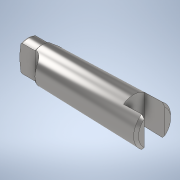
# Autodesk Inventor part: Part005.Morse 5 shaft
Saved by Autodesk Inventor 2022.2 (Build 262287010, 287A)
## iProperties
Created: 2022-11-30
Part Number: Part005.Morse 5 shaft
Material: Steel, Alloy
Document SubType Name: Modeling
Designer: User
Mass: 1240.36 g
Surface Area: 217.832 cm^2
Volume: 160.46 cm^3
Density: 7.73 g/cm^3
Appearance: Semi-Polished
Author: User
Autodesk Inventor part; units mm, degrees
ref_plane "YZ Plane" through (0, 0, 0) normal (1, 0, 0) x (0, 1, 0)
ref_plane "XZ Plane" through (0, 0, 0) normal (0, 1, 0) x (-1, 0, 0)
ref_plane "XY Plane" through (0, 0, 0) normal (0, 0, 1) x (1, 0, 0)
sketch "Sketch1" plane through (0, 0, 0) normal (0, 0, 1) x (1, 0, 0)
  line L0 (0, 0) -> (0, 18.2735) construction
  line L1 (0, 18.2735) -> (20.5646, 18.8146) construction
  line L2 (155.5, 22.3653) -> (155.5, 0)
  line L3 (155.5, 0) -> (0, 0)
  line L4 (149.2, 22.1995) -> (149.2, 0) construction
  line L5 (0, 0) -> (2.3398, 16.0387)
  line L6 (4.3188, 17.75) -> (19.5, 17.75)
  line L7 (19.5, 17.75) -> (20.5646, 18.8146)
  arc A0 (4.3188, 17.75) -> (2.3398, 16.0387) centre (4.3188, 15.75) ccw
  line L8 (20.5646, 18.8146) -> (155.5, 22.3653)
  dimension "d0" = 36.547
  dimension "d1" = 155.5
  dimension "d2" = 44.399
  dimension "d3" = 149.2
  dimension "d4" = 35.5
  dimension "d5" = 45
  dimension "d6" = 19.5
  dimension "d7" = 2
  dimension "d8" = 8.3
  constraints: 18 end point, 3 point on line, 2 parallel, 2 point on circle, 2 tangent, 1 centre point, 1 horizontal, 1 perpendicular, 1 vertical
  measures "d0" diameter of L0.end L3
  measures "d1" distance of L2.end L0.start
  measures "d2" diameter of L4.start L3
  measures "d3" distance between parallel lines of L0 L4
  measures "d4" diameter of L6 L3
  measures "d5" angle of L6 L7
  measures "d6" distance from line of L0 L6.end
  measures "d7" radius of A0
  measures "d8" angle of L5 L0
revolve "Revolution1" add sketch "Sketch1" angle 360 about axis through (155.5, 0, 0) along (-1, 0, 0)
sketch "Sketch2" plane through (0, 0, 0) normal (0, 1, 0) x (-1, 0, 0)
  line L0 (0, 7.95) -> (-19.5007, 7.95)
  arc A0 (-24.5298, 28.7331) -> (-19.5007, 7.95) centre (-19.5007, 18.95) ccw
  line L1 (-24.5298, 28.7331) -> (0, 28.7331)
  line L2 (0, 28.7331) -> (0, 7.95)
  line L3 (31.1, 0) -> (-186.6, 0) projected
  line L4 (-20.5646, 18.8146) -> (-155.5, 22.3653) construction
  point P0 (0, 0)
  point P1 (-30.5, 19.0761)
  dimension "d10" = 15.9
  dimension "d11" = 11
  dimension "d12" = 30.5
  constraints: 6 end point, 3 point on circle, 2 point on line, 1 centre point, 1 horizontal, 1 parallel, 1 perpendicular, 1 tangent
  measures "d10" diameter of L0 L3
  measures "d11" radius of A0
  measures "d12" distance from line of L2 point (-30.5, 19.076)
extrude "Extrusion1" cut sketch "Sketch2" along normal through all both and the other way through all
mirror "Mirror1" about plane through (0, 0, 0) normal (0, 0, 1) of "Extrusion1"
chamfer "Chamfer1" distance 3 angle 45 1 edges at (155.5, -22.3653, 0)
sketch "Sketch3" plane through (0, 0, 0) normal (0, 1, 0) x (-1, 0, 0)
  line L0 (-155.5, 12.5) -> (-130.5, 12.5)
  line L1 (-130.5, 12.5) -> (-130.5, -12.5)
  line L2 (-130.5, -12.5) -> (-155.5, -12.5)
  line L3 (-155.5, -12.5) -> (-155.5, 12.5)
  line L4 (-155.5, -19.3653) -> (-155.5, 19.3653) construction
  point P0 (0, 0)
  point P1 (-155.5, 0)
  dimension "d18" = 25
  dimension "d19" = 25
  constraints: 8 end point, 2 midpoint, 2 parallel, 1 horizontal, 1 perpendicular
  measures "d18" distance between parallel lines of L3 L1
  measures "d19" distance between parallel lines of L2 L0
extrude "Extrusion2" cut sketch "Sketch3" along normal through all both and the other way through all
body "Solid1"
